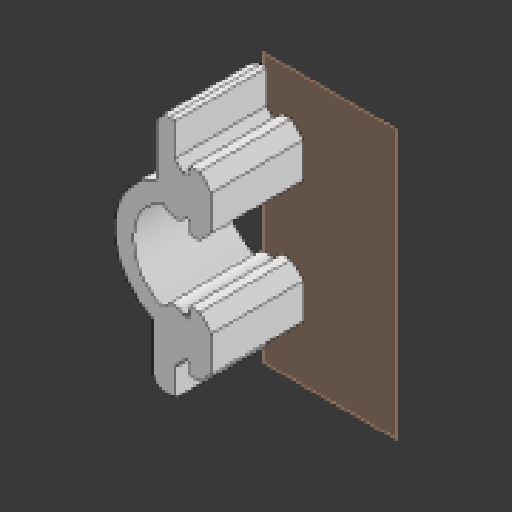
# Autodesk Inventor part: Camera Wire Clip
Saved by Autodesk Inventor 2023 (Build 270158000, 158)
## iProperties
Created: 2023-01-05
Part Number: Camera Wire Clip
Material: Generic
Document SubType Name: Modeling
Designer: alber
Density: 1 g/cm^3
Appearance: Default
Author: alber
Autodesk Inventor part; units mm, degrees
ref_plane "YZ Plane" through (0, 0, 0) normal (1, 0, 0) x (0, 1, 0)
ref_plane "XZ Plane" through (0, 0, 0) normal (0, 1, 0) x (-1, 0, 0)
ref_plane "XY Plane" through (0, 0, 0) normal (0, 0, 1) x (1, 0, 0)
ref_plane "Work Plane1" through (0, 0, 0) normal (0, 0, 1) x (1, 0, 0)
sketch "Sketch1" plane through (0, 0, 0) normal (0, 0, 1) x (1, 0, 0)
  line L0 (-145, -10) -> (145, -10) projected
  line L1 (-10, 38) -> (-10, -12) projected
  line L2 (-123, 38) -> (-10, 38) projected
  line L3 (-123, -12) -> (-123, 38) projected
  line L4 (-123, -12) -> (-10, -12) projected
  line L5 (-2.2716, -121.1355) -> (-2.2716, -6.1355) projected
  line L6 (-8.2, 6.2) -> (-5.2101, 6.2)
  line L7 (-5.2101, 6.2) -> (-3.0101, 4)
  line L8 (-3.0101, 4) -> (-0.5, 4)
  line L9 (-0.5, 4) -> (0, 3.5)
  line L10 (0, 3.5) -> (0.5, 4)
  line L11 (0.5, 4) -> (3.0101, 4)
  line L12 (3.0101, 4) -> (5.2101, 6.2)
  line L13 (5.2101, 6.2) -> (8.2, 6.2)
  line L14 (8.2, 6.2) -> (8.2, 13.8828)
  line L15 (8.2, 13.8828) -> (5.2101, 13.8828)
  line L16 (5.2101, 13.8828) -> (3.0101, 16.0828)
  line L17 (3.0101, 16.0828) -> (0.5, 16.0828)
  line L18 (0.5, 16.0828) -> (0, 16.5828)
  line L19 (0, 16.5828) -> (-0.5, 16.0828)
  line L20 (-0.5, 16.0828) -> (-3.0101, 16.0828)
  line L21 (-3.0101, 16.0828) -> (-5.2101, 13.8828)
  line L22 (-5.2101, 13.8828) -> (-8.2, 13.8828)
  line L23 (-8.2, 13.8828) -> (-8.2, 6.2)
  line L24 (-8.2, 16.6) -> (-8.2, 14.7899)
  line L25 (-8.2, 14.7899) -> (-6.2, 14.7899)
  line L26 (-6.2, 14.7899) -> (-4, 16.9899)
  line L27 (-4, 16.9899) -> (-4, 19.5)
  line L28 (-4, 19.5) -> (-3.5, 20)
  line L29 (-3.5, 20) -> (-4, 20.5)
  line L30 (-4, 20.5) -> (-4, 23.0101)
  line L31 (-4, 23.0101) -> (-6.2, 25.2101)
  line L32 (-6.2, 25.2101) -> (-8.2, 25.2101)
  line L33 (-8.2, 25.2101) -> (-8.2, 23)
  line L34 (-8.2, 23) -> (-10, 24.8)
  line L35 (-10, 24.8) -> (-10, 30)
  line L36 (-9.0101, 30) -> (-4.8, 30)
  line L37 (-4.8, 30) -> (-3, 28.2)
  line L38 (-3, 28.2) -> (-5.2101, 28.2)
  line L39 (-5.2101, 28.2) -> (-5.2101, 26.2)
  line L40 (-5.2101, 26.2) -> (-3.0101, 24)
  line L41 (-3.0101, 24) -> (-0.5, 24)
  line L42 (-0.5, 24) -> (0, 23.5)
  line L43 (0, 23.5) -> (0.5, 24)
  line L44 (0.5, 24) -> (3.0101, 24)
  line L45 (3.0101, 24) -> (5.2101, 26.2)
  line L46 (5.2101, 26.2) -> (5.2101, 28.2)
  line L47 (5.2101, 28.2) -> (3, 28.2)
  line L48 (3, 28.2) -> (4.8, 30)
  line L49 (4.8, 30) -> (10, 30)
  line L50 (10, 30) -> (10, 24.8)
  line L51 (10, 24.8) -> (8.2, 23)
  line L52 (8.2, 23) -> (8.2, 25.2101)
  line L53 (8.2, 25.2101) -> (6.2, 25.2101)
  line L54 (6.2, 25.2101) -> (4, 23.0101)
  line L55 (4, 23.0101) -> (4, 20.5)
  line L56 (4, 20.5) -> (3.5, 20)
  line L57 (3.5, 20) -> (4, 19.5)
  line L58 (4, 19.5) -> (4, 16.9899)
  line L59 (4, 16.9899) -> (6.2, 14.7899)
  line L60 (6.2, 14.7899) -> (8.2, 14.7899)
  line L61 (8.2, 14.7899) -> (8.2, 17)
  line L62 (8.2, 17) -> (10, 15.2)
  line L63 (10, 15.2) -> (10, 4.8828)
  arc A0 (9.9414, 4.7414) -> (10, 4.8828) centre (9.8, 4.8828) ccw
  line L64 (9.9414, 4.7414) -> (8.5414, 3.3414)
  arc A1 (8.2, 3.4828) -> (8.5414, 3.3414) centre (8.4, 3.4828) ccw
  line L65 (8.2, 3.4828) -> (8.2, 5.2101)
  line L66 (8.2, 5.2101) -> (6.2, 5.2101)
  line L67 (6.2, 5.2101) -> (4, 3.0101)
  line L68 (4, 3.0101) -> (4, 0.5)
  line L69 (4, 0.5) -> (3.5, 0)
  line L70 (3.5, 0) -> (4, -0.5)
  line L71 (4, -0.5) -> (4, -3.0101)
  line L72 (4, -3.0101) -> (6.2, -5.2101)
  line L73 (6.2, -5.2101) -> (8.2, -5.2101)
  line L74 (8.2, -5.2101) -> (8.2, -3.4828)
  arc A2 (8.5414, -3.3414) -> (8.2, -3.4828) centre (8.4, -3.4828) ccw
  line L75 (8.5414, -3.3414) -> (9.9414, -4.7414)
  arc A3 (10, -4.8828) -> (9.9414, -4.7414) centre (9.8, -4.8828) ccw
  line L76 (10, -4.8828) -> (10, -9.8)
  arc A4 (9.8, -10) -> (10, -9.8) centre (9.8, -9.8) ccw
  line L77 (9.8, -10) -> (4.8828, -10)
  arc A5 (4.7414, -9.9414) -> (4.8828, -10) centre (4.8828, -9.8) ccw
  line L78 (4.7414, -9.9414) -> (3.3414, -8.5414)
  arc A6 (3.4828, -8.2) -> (3.3414, -8.5414) centre (3.4828, -8.4) ccw
  line L79 (3.4828, -8.2) -> (5.2101, -8.2)
  line L80 (5.2101, -8.2) -> (5.2101, -6.2)
  line L81 (5.2101, -6.2) -> (3.0101, -4)
  line L82 (3.0101, -4) -> (0.5, -4)
  line L83 (0.5, -4) -> (0, -3.5)
  line L84 (0, -3.5) -> (-0.5, -4)
  line L85 (-0.5, -4) -> (-3.0101, -4)
  line L86 (-3.0101, -4) -> (-5.2101, -6.2)
  line L87 (-5.2101, -6.2) -> (-5.2101, -8.2)
  line L88 (-5.2101, -8.2) -> (-3.4828, -8.2)
  arc A7 (-3.3414, -8.5414) -> (-3.4828, -8.2) centre (-3.4828, -8.4) ccw
  line L89 (-3.3414, -8.5414) -> (-4.7414, -9.9414)
  arc A8 (-4.8828, -10) -> (-4.7414, -9.9414) centre (-4.8828, -9.8) ccw
  line L90 (-10, -9.8) -> (-10, -4.8828)
  arc A9 (-9.9414, -4.7414) -> (-10, -4.8828) centre (-9.8, -4.8828) ccw
  line L91 (-9.9414, -4.7414) -> (-8.5414, -3.3414)
  arc A10 (-8.2, -3.4828) -> (-8.5414, -3.3414) centre (-8.4, -3.4828) ccw
  line L92 (-8.2, -3.4828) -> (-8.2, -5.2101)
  line L93 (-8.2, -5.2101) -> (-6.2, -5.2101)
  line L94 (-6.2, -5.2101) -> (-4, -3.0101)
  line L95 (-4, -3.0101) -> (-4, -0.5)
  line L96 (-4, -0.5) -> (-3.5, 0)
  line L97 (-3.5, 0) -> (-4, 0.5)
  line L98 (-4, 0.5) -> (-4, 3.0101)
  line L99 (-4, 3.0101) -> (-6.2, 5.2101)
  line L100 (-6.2, 5.2101) -> (-8.2, 5.2101)
  line L101 (-8.2, 5.2101) -> (-8.2, 3.4828)
  arc A11 (-8.5414, 3.3414) -> (-8.2, 3.4828) centre (-8.4, 3.4828) ccw
  line L102 (-8.5414, 3.3414) -> (-9.9414, 4.7414)
  arc A12 (-10, 4.8828) -> (-9.9414, 4.7414) centre (-9.8, 4.8828) ccw
  line L103 (-10, 4.8828) -> (-10, 15.2)
  line L104 (-10, 15.2) -> (-8.4, 16.8)
  arc A13 (-8.2, 16.6) -> (-8.4, 16.8) centre (-8.4, 16.6) ccw
  circle A14 centre (0, 20) radius 2
  circle A15 centre (0, 0) radius 2
  line L105 (-4.8828, -10) -> (-8.2, -10)
  line L106 (-10.3707, 24.6827) -> (-7.8549, 22.1669)
  line L107 (-7.8549, 22.1669) -> (-7.8549, 24.865)
  line L108 (-7.8549, 24.865) -> (-6.3429, 24.865)
  line L109 (-6.3429, 24.865) -> (-4.3451, 22.8671)
  line L110 (-4.3451, 22.8671) -> (-4.3451, 20.2929)
  line L111 (-4.3451, 19.7071) -> (-4.3451, 17.1329)
  line L112 (-4.3451, 17.1329) -> (-6.3429, 15.135)
  line L113 (-6.3429, 15.135) -> (-7.8549, 15.135)
  line L114 (-7.8549, 15.135) -> (-7.8549, 16.6)
  arc A16 (-7.8549, 16.6) -> (-8.7381, 17.0275) centre (-8.4, 16.6) ccw
  line L115 (-8.7381, 17.0275) -> (-10.3707, 15.395)
  line L116 (-10.3, 4.6757) -> (-8.7536, 3.1293)
  arc A17 (-8.7536, 3.1293) -> (-7.9, 3.4828) centre (-8.4, 3.4828) ccw
  line L117 (-7.9, 3.4828) -> (-7.9, 4.9101)
  line L118 (-7.9, 4.9101) -> (-6.3243, 4.9101)
  line L119 (-6.3243, 4.9101) -> (-4.3, 2.8858)
  line L120 (-4.3, 2.8858) -> (-4.3, 0.2929)
  line L121 (-4.3, -0.2929) -> (-4.3, -2.8858)
  line L122 (-4.3, -2.8858) -> (-6.3243, -4.9101)
  line L123 (-6.3243, -4.9101) -> (-7.9, -4.9101)
  line L124 (-7.9, -4.9101) -> (-7.9, -3.4828)
  arc A18 (-7.9, -3.4828) -> (-8.7536, -3.1293) centre (-8.4, -3.4828) ccw
  line L125 (-8.7536, -3.1293) -> (-10.1536, -4.5293)
  arc A19 (-10.1536, -4.5293) -> (-10.3, -4.8828) centre (-9.8, -4.8828) ccw
  line L126 (-10.3, -4.8828) -> (-10.3, -9.2902)
  line L127 (-4.3451, 19.7071) -> (-4.3451, 20.2929)
  line L128 (-4.3, -0.2929) -> (-4.3, 0.2929)
  line L129 (-10.3, -9.2902) -> (-13.9747, -9.2902)
  line L130 (-13.3707, 30.0707) -> (-10.3707, 30.0707)
  line L131 (-145, 15.1172) -> (-1.076, 15.1172) projected
  line L132 (-10.3707, 30.0707) -> (-10.3707, 15.395)
  line L133 (-10.3, 4.6757) -> (-10.3, -9.2902)
  line L134 (-10.3, 15.1172) -> (-10.3, 15.135)
  line L135 (-13.9747, -9.2902) -> (-13.9747, 0.0372)
  arc A20 (-12.3822, 17.4064) -> (-12.3746, 2.6011) centre (-9.1048, 10.0054) ccw
  arc A21 (-13.3707, 20.2467) -> (-13.9747, 0.0372) centre (-9.1048, 10.0054) ccw
  line L136 (-13.3707, 16.8707) -> (-13.3707, 16.8842)
  line L137 (-13.3707, 20.2467) -> (-13.3707, 30.0707)
  line L138 (-10.3707, 15.395) -> (-12.3822, 17.4064)
  line L139 (-10.3707, 15.395) -> (-8.2646, 15.395) construction
  line L140 (-10.3, 4.6757) -> (-12.3746, 2.6011)
  line L141 (-10.3, 4.6757) -> (-7.366, 4.6757) construction
  point P0 (0, 0)
  point P1 (-9.8, -10)
  point P2 (-10.2243, 4.6)
  point P3 (-13.9747, 3.5401)
  point P4 (-10.3, 24.6757)
  point P5 (-10.3, -4.8828)
  point P6 (-10.3, -4.8828)
  dimension "d0" = 0.4
  dimension "d1" = 3
  dimension "d13" = 3
  dimension "d14" = 135
  dimension "d15" = 135
  constraints: 270 end point, 42 point on circle, 31 horizontal, 30 vertical, 22 centre point, 7 parallel, 7 point on line, 3 perpendicular, 1 equal length, 209 other
  measures "d0" distance between parallel lines of L104 L115
  measures "d1" distance of L130.start L130.end
  measures "d13" radial gap between concentric circles of A20 A21
  measures "d14" angle of L139 L138
  measures "d15" angle of L140 L141
extrude "Extrusion1" add sketch "Sketch1" along normal blind 15 contours A21 L137 L130 L132 L138 A20 L131 | L131 A20 L140 L133 L126 L129 L135 A21 | L125 A19 L133 L116 L1 | L1 L116 A17 L117 L118 L119 L120 L128 L121 L122 L123 L124 A18 L125 | L106 L107 L108 L109 L110 L127 L111 L112 L113 L114 A16 L115 L1 | L1 L115 L132 L106
fillet "Fillet1" radius 0.7 1 edges at (-7.8549, 22.1669, 7.5)
fillet "Fillet2" radius 2 2 edges at (-13.9747, -9.2902, 7.5) (-13.3707, 30.0707, 7.5)
fillet "Fillet3" radius 2 2 edges at (-10.3, 4.6757, 7.5) (-10.3707, 15.395, 7.5)
body "Solid1"
